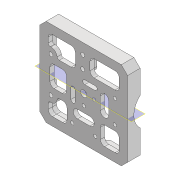
# Autodesk Inventor part: base_shell_2
Saved by Autodesk Inventor 2020 (Build 240168000, 168)
## iProperties
Created: 2022-01-22
Part Number: base_shell_2
Material: Generic
Document SubType Name: Modeling
Designer: Shuang Peng
Density: 1 g/cm^3
Appearance: Default
Author: Shuang Peng
Autodesk Inventor part; units mm, degrees
ref_plane "YZ Plane" through (0, 0, 0) normal (1, 0, 0) x (0, 1, 0)
ref_plane "XZ Plane" through (0, 0, 0) normal (0, 1, 0) x (-1, 0, 0)
ref_plane "XY Plane" through (0, 0, 0) normal (0, 0, 1) x (1, 0, 0)
sketch "Sketch1" plane through (0, 0, 0) normal (0, 0, 1) x (1, 0, 0)
  circle A0 centre (7.5, 4) radius 0.75 projected
  circle A1 centre (13, -5.9) radius 0.75 projected
  circle A2 centre (2, -5.9) radius 0.75 projected
  line L0 (15, -7) -> (15, 0) projected
  line L1 (11, 0) -> (15, 0) projected
  arc A3 (10, 1) -> (11, 0) centre (11, 1) ccw projected
  line L2 (10, 1) -> (10, 5) projected
  line L3 (6, 6) -> (9, 6) projected
  line L4 (5, 1) -> (5, 5) projected
  arc A4 (4, 0) -> (5, 1) centre (4, 1) ccw projected
  line L5 (0, 0) -> (4, 0) projected
  line L6 (0, -7) -> (0, 0) projected
  line L7 (1.5, -8.5) -> (5, -8.5) projected
  line L8 (13, -5.9) -> (2, -5.9)
  line L9 (7.5, -5.9) -> (7.5, -9.9)
  line L10 (7.5, -9.9) -> (-2.5, -9.9)
  line L11 (-23.5, -30.9) -> (-23.5, 11.1)
  line L12 (-23.5, 11.1) -> (18.5, 11.1)
  line L13 (18.5, 11.1) -> (18.5, -30.9)
  line L14 (18.5, -30.9) -> (-23.5, -30.9)
  line L15 (-23.5, -30.9) -> (18.5, 11.1) construction
  line L16 (-23.5, 11.1) -> (18.5, -30.9) construction
  circle A5 centre (-15.2, -15.4) radius 0.75 projected
  circle A6 centre (-15.2, -4.4) radius 0.75 projected
  circle A7 centre (-15.2, -15.4) radius 0.85
  circle A8 centre (-15.2, -4.4) radius 0.85
  circle A9 centre (-5.3, -9.9) radius 0.75 projected
  circle A10 centre (-5.3, -9.9) radius 0.85
  circle A11 centre (2, -5.9) radius 0.85
  circle A12 centre (13, -5.9) radius 0.85
  circle A13 centre (7.5, 4) radius 0.85
  line L17 (6, -7.5) -> (6, -4.5) projected
  arc A14 (9, -4.5) -> (6, -4.5) centre (7.5, -4.5) ccw projected
  line L18 (9, -4.5) -> (9, -7.5) projected
  line L19 (10, -8.5) -> (13.5, -8.5) projected
  arc A15 (6, 6) -> (5, 5) centre (6, 5) ccw projected
  line L20 (1.5, -8.5) -> (0, -7) projected
  arc A16 (5, -8.5) -> (6, -7.5) centre (5, -7.5) ccw projected
  arc A17 (9, -7.5) -> (10, -8.5) centre (10, -7.5) ccw projected
  line L21 (15, -7) -> (13.5, -8.5) projected
  arc A18 (10, 5) -> (9, 6) centre (9, 5) ccw projected
  dimension "d0" = 4
  dimension "d1" = 10
  dimension "d2" = 42
  dimension "d3" = 42
  dimension "d4" = 1.7
  dimension "d5" = 1.7
  dimension "d6" = 1.7
  dimension "d7" = 1.7
  dimension "d8" = 1.7
  dimension "d9" = 1.7
  constraints: 18 end point, 6 centre point, 6 coincident, 3 midpoint, 3 perpendicular, 2 parallel, 1 horizontal, 1 vertical
  measures "d0" distance of L9.start L9.end
  measures "d1" distance of L9.end L10.end
  measures "d2" distance of L11.start L11.end
  measures "d3" distance of L11.end L12.end
  measures "d4" diameter of A7
  measures "d5" diameter of A8
  measures "d6" diameter of A10
  measures "d7" diameter of A11
  measures "d8" diameter of A12
  measures "d9" diameter of A13
extrude "Extrusion1" add sketch "Sketch1" along normal blind 2 contours L21 L19 A17 L18 A14 L17 A16 L7 L20 L6 L5 A4 L4 A15 L3 A18 L2 A3 L1 L0 | L8 L17 A14 L18 | L11 L12 L13 L14
sketch "Sketch2" plane through (0, 0, 0) normal (0, 0, -1) x (-1, 0, 0)
  line L0 (23.5, -30.9) -> (-18.5, -30.9) projected
  line L1 (23.5, 11.1) -> (23.5, -30.9) projected
  line L2 (-18.5, 11.1) -> (23.5, 11.1) projected
  line L3 (-18.5, -30.9) -> (-18.5, 11.1) projected
  circle A0 centre (-2, -5.9) radius 0.85 projected
  circle A1 centre (15.2, -15.4) radius 0.85 projected
  circle A2 centre (15.2, -4.4) radius 0.85 projected
  circle A3 centre (5.3, -9.9) radius 0.85 projected
  circle A4 centre (-13, -5.9) radius 0.85 projected
  circle A5 centre (-7.5, 4) radius 0.85 projected
  line L4 (23.5, -30.9) -> (-18.5, -30.9) projected
  line L5 (-18.5, -30.9) -> (23.5, 11.1)
  line L6 (23.5, -30.9) -> (-18.5, 11.1)
  line L7 (-16.5, -28.9) -> (-16.5, 9.1)
  line L8 (-16.5, 9.1) -> (21.5, 9.1)
  line L9 (21.5, 9.1) -> (21.5, -28.9)
  line L10 (21.5, -28.9) -> (-16.5, -28.9)
  line L11 (-16.5, -28.9) -> (21.5, 9.1) construction
  line L12 (-16.5, 9.1) -> (21.5, -28.9) construction
  point P0 (0, 0)
  point P1 (2.5, -9.9)
  dimension "d12" = 38
  dimension "d13" = 38
  constraints: 16 end point, 3 midpoint, 2 parallel, 1 perpendicular, 1 vertical
  measures "d12" distance of L8.end L9.end
  measures "d13" distance of L7.end L8.end
extrude "Extrusion2" add sketch "Sketch2" along normal blind 4 contours L6 L9 L5 L1 | L0 L5 L10 L6 | L3 L6 L7 L5 | L5 L8 L6 L2
fillet "Fillet1" radius 2 1 edges at (16.5, -28.9, -2)
sketch "Sketch4" plane through (-23.5, -30.9, 2) normal (-1, 0, 0) x (0, 0, 1)
  circle A0 centre (-12, 21) radius 0.75 projected
  circle A1 centre (-12, 21) radius 9
  point P0 (-2, 30.9)
  dimension "d21" = 18
  constraints: 1 centre point, 1 coincident
  measures "d21" diameter of A1
extrude "Extrusion4" cut sketch "Sketch4" against normal blind 4
chamfer "Chamfer1" distance 3 angle 45 4 edges at (-23.5, -30.9, -1) (-23.5, 11.1, -1) (18.5, 11.1, -1) (18.5, -30.9, -1)
sketch "Sketch8" plane through (0, 0, 0) normal (0, 0, -1) x (-1, 0, 0)
  circle A0 centre (-2, -5.9) radius 0.85 projected
  circle A1 centre (15.2, -15.4) radius 0.85 projected
  circle A2 centre (15.2, -4.4) radius 0.85 projected
  circle A3 centre (5.3, -9.9) radius 0.85 projected
  circle A4 centre (-13, -5.9) radius 0.85 projected
  circle A5 centre (-7.5, 4) radius 0.85 projected
  line L0 (15.2, -4.4) -> (18.2, -4.4)
  line L1 (18.2, -4.4) -> (18.2, -1.4)
  line L2 (15.2, -15.4) -> (18.2, -15.4)
  line L3 (18.2, -15.4) -> (18.2, -18.4)
  circle A6 centre (18.2, -1.4) radius 0.95
  circle A7 centre (18.2, -18.4) radius 0.95
  line L4 (-14.5, -28.9) -> (21.5, -28.9) projected
  line L5 (21.5, -28.9) -> (21.5, 9.1) projected
  line L6 (21.5, 9.1) -> (-16.5, 9.1) projected
  line L7 (-16.5, 9.1) -> (-16.5, -26.9) projected
  arc A8 (-16.5, -26.9) -> (-14.5, -28.9) centre (-14.5, -26.9) ccw projected
  point P0 (0, 0)
  dimension "d53" = 3
  dimension "d54" = 3
  dimension "d55" = 3
  dimension "d56" = 3
  dimension "d57" = 1.9
  dimension "d58" = 1.9
  constraints: 8 end point, 2 centre point, 2 coincident, 2 horizontal, 2 perpendicular
  measures "d53" distance of L0.start L0.end
  measures "d54" distance of L0.end L1.end
  measures "d55" distance of L2.start L2.end
  measures "d56" distance of L2.end L3.end
  measures "d57" diameter of A6
  measures "d58" diameter of A7
extrude "Extrusion8" cut sketch "Sketch8" against normal blind 4 contours A6 | A7
sketch "Sketch9" plane through (0, 0, 0) normal (0, 0, -1) x (-1, 0, 0)
  circle A0 centre (18.2, -18.4) radius 0.95 projected
  circle A1 centre (18.2, -1.4) radius 0.95 projected
  circle A2 centre (-2, -5.9) radius 0.85 projected
  circle A3 centre (15.2, -15.4) radius 0.85 projected
  circle A4 centre (15.2, -4.4) radius 0.85 projected
  circle A5 centre (5.3, -9.9) radius 0.85 projected
  circle A6 centre (-13, -5.9) radius 0.85 projected
  circle A7 centre (-7.5, 4) radius 0.85 projected
  line L0 (0, 0) -> (3, 0)
  line L1 (3, 0) -> (3, 6)
  circle A8 centre (3, 6) radius 0.95
  circle A9 centre (3, 0) radius 0.95
  line L2 (-14.5, -28.9) -> (21.5, -28.9) projected
  line L3 (21.5, -28.9) -> (21.5, 9.1) projected
  line L4 (21.5, 9.1) -> (-16.5, 9.1) projected
  line L5 (-16.5, 9.1) -> (-16.5, -26.9) projected
  arc A10 (-16.5, -26.9) -> (-14.5, -28.9) centre (-14.5, -26.9) ccw projected
  dimension "d61" = 3
  dimension "d62" = 6
  dimension "d63" = 1.9
  dimension "d64" = 1.9
  constraints: 4 end point, 2 centre point, 2 coincident, 1 horizontal, 1 vertical
  measures "d61" distance of L0.start L0.end
  measures "d62" distance of L0.end L1.end
  measures "d63" diameter of A8
  measures "d64" diameter of A9
extrude "Extrusion9" cut sketch "Sketch9" against normal blind 4 contours A9 L1 L0 | L0 L1 A9 | A8
sketch "Sketch10" plane through (0, 0, 0) normal (0, 0, -1) x (-1, 0, 0)
  circle A0 centre (3, 0) radius 0.95 projected
  circle A1 centre (3, 6) radius 0.95 projected
  circle A2 centre (18.2, -18.4) radius 0.95 projected
  circle A3 centre (18.2, -1.4) radius 0.95 projected
  circle A4 centre (-2, -5.9) radius 0.85 projected
  circle A5 centre (15.2, -15.4) radius 0.85 projected
  circle A6 centre (15.2, -4.4) radius 0.85 projected
  circle A7 centre (5.3, -9.9) radius 0.85 projected
  circle A8 centre (-13, -5.9) radius 0.85 projected
  circle A9 centre (-7.5, 4) radius 0.85 projected
  line L0 (3, 0) -> (3, 6) construction
  line L1 (5.3, 0) -> (5.3, 6)
  line L2 (0.7, 6) -> (0.7, 0)
  arc A10 (0.7, 0) -> (5.3, 0) centre (3, 0) ccw
  arc A11 (5.3, 6) -> (0.7, 6) centre (3, 6) ccw
  line L3 (0.7, 6) -> (5.3, 6)
  line L4 (5.3, 6) -> (5.3, 10)
  line L5 (5.3, 10) -> (0.7, 10)
  line L6 (0.7, 10) -> (0.7, 6)
  line L7 (-14.5, -28.9) -> (21.5, -28.9) projected
  line L8 (21.5, -28.9) -> (21.5, 9.1) projected
  line L9 (21.5, 9.1) -> (-16.5, 9.1) projected
  line L10 (-16.5, 9.1) -> (-16.5, -26.9) projected
  arc A12 (-16.5, -26.9) -> (-14.5, -28.9) centre (-14.5, -26.9) ccw projected
  point P0 (0, 0)
  point P1 (3, 3)
  dimension "d67" = 4.6
  dimension "d68" = 4.6
  dimension "d69" = 4
  constraints: 16 end point, 4 point on circle, 4 tangent, 3 parallel, 2 centre point, 1 horizontal, 1 midpoint, 1 perpendicular, 1 vertical
  measures "d67" diameter of A11
  measures "d68" distance of L5.end L4.end
  measures "d69" distance of L4.end L3.end
extrude "Extrusion10" add sketch "Sketch10" along normal blind 2.5 contours L3 L1 A10 L2 A1 | A1 L3 A11 | A11 L6 L9 L4 | L9 L6 L5 L4
sketch "Sketch11" plane through (0, 0, 0) normal (0, 0, -1) x (-1, 0, 0)
  circle A0 centre (-7.5, 4) radius 0.85 projected
  circle A1 centre (-13, -5.9) radius 0.85 projected
  circle A2 centre (5.3, -9.9) radius 0.85 projected
  circle A3 centre (15.2, -4.4) radius 0.85 projected
  circle A4 centre (15.2, -15.4) radius 0.85 projected
  circle A5 centre (-2, -5.9) radius 0.85 projected
  line L0 (5.3, 9.1) -> (5.3, 0) projected
  arc A6 (0.7, 0) -> (5.3, 0) centre (3, 0) ccw projected
  line L1 (0.7, 0) -> (0.7, 9.1) projected
  line L2 (0.7, 9.1) -> (-16.5, 9.1) projected
  line L3 (-16.5, 9.1) -> (-16.5, -26.9) projected
  arc A7 (-16.5, -26.9) -> (-14.5, -28.9) centre (-14.5, -26.9) ccw projected
  line L4 (-14.5, -28.9) -> (21.5, -28.9) projected
  line L5 (21.5, -28.9) -> (21.5, 9.1) projected
  line L6 (21.5, 9.1) -> (5.3, 9.1) projected
  circle A8 centre (18.2, -1.4) radius 0.95 projected
  circle A9 centre (18.2, -18.4) radius 0.95 projected
  point P0 (0, 0)
extrude "Extrusion11" add sketch "Sketch11" against normal up to surface (2 mm away) contours A0 | A1 | A2 | A3 | A4 | A5
sketch "Sketch12" plane through (0, 0, 2) normal (0, 0, 1) x (1, 0, 0)
  arc A0 (0.5, -11.4) -> (1.5, -12.4) centre (1.5, -11.4) ccw projected
  line L0 (5, -12.4) -> (1.5, -12.4) projected
  arc A1 (6.5, -13.9) -> (5, -12.4) centre (5, -13.9) ccw projected
  line L1 (6.5, -17.4) -> (6.5, -13.9) projected
  line L2 (13.5, -17.4) -> (6.5, -17.4) projected
  line L3 (15, -15.9) -> (13.5, -17.4) projected
  line L4 (15, -15.9) -> (15, -12.4) projected
  arc A2 (15, -12.4) -> (14, -11.4) centre (14, -12.4) ccw projected
  line L5 (14, -11.4) -> (11, -11.4) projected
  arc A3 (11, -8.4) -> (11, -11.4) centre (11, -9.9) ccw projected
  line L6 (11, -8.4) -> (14, -8.4) projected
  arc A4 (14, -8.4) -> (15, -7.4) centre (14, -7.4) ccw projected
  line L7 (15, -7.4) -> (15, -3.9) projected
  line L8 (13.5, -2.4) -> (15, -3.9) projected
  line L9 (13.5, -2.4) -> (6.5, -2.4) projected
  line L10 (6.5, -5.9) -> (6.5, -2.4) projected
  arc A5 (5, -7.4) -> (6.5, -5.9) centre (5, -5.9) ccw projected
  line L11 (5, -7.4) -> (1.5, -7.4) projected
  arc A6 (1.5, -7.4) -> (0.5, -8.4) centre (1.5, -8.4) ccw projected
  line L12 (0.5, -11.4) -> (0.5, -8.4) projected
  circle A7 centre (12.4, -15.4) radius 0.725 projected
  circle A8 centre (12.4, -4.4) radius 0.725 projected
  circle A9 centre (2.5, -9.9) radius 0.725 projected
  arc A10 (-4, -12.9) -> (-5, -13.9) centre (-4, -13.9) ccw projected
  line L13 (-5, -17.4) -> (-5, -13.9) projected
  arc A11 (-6.5, -18.9) -> (-5, -17.4) centre (-6.5, -17.4) ccw projected
  line L14 (-10, -18.9) -> (-6.5, -18.9) projected
  line L15 (-10, -25.9) -> (-10, -18.9) projected
  line L16 (-8.5, -27.4) -> (-10, -25.9) projected
  line L17 (-8.5, -27.4) -> (-5, -27.4) projected
  arc A12 (-5, -27.4) -> (-4, -26.4) centre (-5, -26.4) ccw projected
  line L18 (-4, -26.4) -> (-4, -23.4) projected
  arc A13 (-1, -23.4) -> (-4, -23.4) centre (-2.5, -23.4) ccw projected
  line L19 (-1, -23.4) -> (-1, -26.4) projected
  arc A14 (-1, -26.4) -> (0, -27.4) centre (0, -26.4) ccw projected
  line L20 (0, -27.4) -> (3.5, -27.4) projected
  line L21 (5, -25.9) -> (3.5, -27.4) projected
  line L22 (5, -25.9) -> (5, -18.9) projected
  line L23 (1.5, -18.9) -> (5, -18.9) projected
  arc A15 (0, -17.4) -> (1.5, -18.9) centre (1.5, -17.4) ccw projected
  line L24 (0, -17.4) -> (0, -13.9) projected
  arc A16 (0, -13.9) -> (-1, -12.9) centre (-1, -13.9) ccw projected
  line L25 (-4, -12.9) -> (-1, -12.9) projected
  circle A17 centre (-8, -24.8) radius 0.725 projected
  circle A18 centre (3, -24.8) radius 0.725 projected
  circle A19 centre (-2.5, -14.9) radius 0.725 projected
  point P0 (0, 0)
hole "Hole1" at (12.4, -4.4, 2) at (12.4, -15.4, 2) at (2.5, -9.9, 2) at (-2.5, -14.9, 2) at (-8, -24.8, 2) at (3, -24.8, 2) direction (0, 0, -1) diameter 1.6 depth 10
sketch "Sketch13" plane through (0, 0, 2) normal (0, 0, 1) x (1, 0, 0)
  circle A0 centre (-8, -24.8) radius 0.8 projected
  circle A1 centre (2.5, -9.9) radius 0.8 projected
  circle A2 centre (12.4, -4.4) radius 0.8 projected
  circle A3 centre (12.4, -15.4) radius 0.8 projected
  circle A4 centre (-2.5, -14.9) radius 0.8 projected
  circle A5 centre (3, -24.8) radius 0.8 projected
  circle A6 centre (-3, 0) radius 0.95 projected
  circle A7 centre (-3, 6) radius 0.95 projected
  circle A8 centre (-18.2, -18.4) radius 0.95 projected
  circle A9 centre (-18.2, -1.4) radius 0.95 projected
  line L0 (18.5, -27.9) -> (15.5, -30.9) projected
  line L1 (18.5, -27.9) -> (18.5, 8.1) projected
  line L2 (15.5, 11.1) -> (18.5, 8.1) projected
  line L3 (15.5, 11.1) -> (-20.5, 11.1) projected
  line L4 (-23.5, 8.1) -> (-20.5, 11.1) projected
  line L5 (-23.5, 8.1) -> (-23.5, -27.9) projected
  line L6 (-20.5, -30.9) -> (-23.5, -27.9) projected
  line L7 (-20.5, -30.9) -> (15.5, -30.9) projected
  circle A10 centre (12.4, -4.4) radius 0.8 projected
  line L8 (12.4, -4.4) -> (12.4, -15.4)
  circle A11 centre (2.5, -9.9) radius 0.8 projected
  line L9 (2.5, -9.9) -> (12.4, -9.9)
  line L10 (7.45, -6.9) -> (7.45, -12.9) construction
  line L11 (5.45, -6.9) -> (5.45, -12.9)
  line L12 (9.45, -12.9) -> (9.45, -6.9)
  arc A12 (9.45, -6.9) -> (5.45, -6.9) centre (7.45, -6.9) ccw
  arc A13 (5.45, -12.9) -> (9.45, -12.9) centre (7.45, -12.9) ccw
  circle A14 centre (3, -24.8) radius 0.8 projected
  circle A15 centre (-8, -24.8) radius 0.8 projected
  line L13 (3, -24.8) -> (-8, -24.8)
  circle A16 centre (-2.5, -14.9) radius 0.8 projected
  line L14 (-2.5, -14.9) -> (-2.5, -24.8)
  line L15 (0.5, -19.85) -> (-5.5, -19.85) construction
  line L16 (0.5, -17.85) -> (-5.5, -17.85)
  line L17 (-5.5, -21.85) -> (0.5, -21.85)
  arc A17 (0.5, -21.85) -> (0.5, -17.85) centre (0.5, -19.85) ccw
  arc A18 (-5.5, -17.85) -> (-5.5, -21.85) centre (-5.5, -19.85) ccw
  point P0 (0, 0)
  point P1 (7.45, -9.9)
  point P2 (-2.5, -19.85)
  dimension "d82" = 3
  dimension "d83" = 4
  dimension "d84" = 3
  dimension "d85" = 4
  constraints: 24 end point, 8 point on circle, 8 tangent, 6 midpoint, 4 centre point, 2 parallel, 2 perpendicular, 1 horizontal, 1 vertical
  measures "d82" distance of point (7.45, -9.9) L10.end
  measures "d83" diameter of A13
  measures "d84" distance of point (-2.5, -19.85) L15.end
  measures "d85" diameter of A18
extrude "Extrusion12" cut sketch "Sketch13" against normal blind 10 contours L11 A12 L12 L9 | L9 L12 A13 L11 | L16 A17 L17 L14 | L14 L17 A18 L16
sketch "Sketch14" plane through (18.5, -27.9, -4) normal (1, 0, 0) x (0, 0, -1)
  circle A0 centre (6, 18) radius 1 projected
  circle A1 centre (6, 18) radius 9
  line L0 (0, 0) -> (-6, 0) projected
  line L1 (0, 36) -> (0, 0) projected
  line L2 (-6, 36) -> (0, 36) projected
  line L3 (-6, 0) -> (-6, 36) projected
  point P0 (-4, 27.9)
  point P1 (0, 11.2918)
  point P2 (0, 24.7082)
  dimension "d88" = 18
  constraints: 1 centre point, 1 coincident
  measures "d88" diameter of A1
extrude "Extrusion13" cut sketch "Sketch14" against normal blind 10 contours L1 A1 picked at (-0.4747, 16.3042)
sketch "Sketch15" plane through (-20.5, -30.9, 2) normal (0, -1, 0) x (1, 0, 0)
  line L0 (36, 0) -> (36, -6) projected
  line L1 (0, 0) -> (36, 0) projected
  line L2 (0, -6) -> (0, 0) projected
  line L3 (36, -6) -> (0, -6) projected
  circle A0 centre (18, -12) radius 1 projected
  circle A1 centre (18, -12) radius 9
  point P0 (20.5, -2)
  point P1 (11.2918, -6)
  point P2 (24.7082, -6)
  dimension "d91" = 18
  constraints: 1 centre point, 1 coincident
  measures "d91" diameter of A1
extrude "Extrusion14" cut sketch "Sketch15" against normal blind 10 contours L3 A1 picked at (17.6404, -5.0216)
fillet "Fillet5" radius 2 3 edges at (-21.5, 9.1, -2) (-21.5, -28.9, -2) (16.5, 9.1, -2)
sketch "Sketch16" plane through (0, 0, 0) normal (0, 0, -1) x (-1, 0, 0)
  arc A0 (-14.5, 9.1) -> (-16.5, 7.1) centre (-14.5, 7.1) ccw projected
  line L0 (-16.5, 7.1) -> (-16.5, -26.9) projected
  arc A1 (-16.5, -26.9) -> (-14.5, -28.9) centre (-14.5, -26.9) ccw projected
  line L1 (-14.5, -28.9) -> (19.5, -28.9) projected
  arc A2 (19.5, -28.9) -> (21.5, -26.9) centre (19.5, -26.9) ccw projected
  line L2 (21.5, -26.9) -> (21.5, 7.1) projected
  arc A3 (21.5, 7.1) -> (19.5, 9.1) centre (19.5, 7.1) ccw projected
  line L3 (19.5, 9.1) -> (5.3, 9.1) projected
  line L4 (5.3, 9.1) -> (5.3, 0) projected
  arc A4 (0.7, 0) -> (5.3, 0) centre (3, 0) ccw projected
  line L5 (0.7, 0) -> (0.7, 9.1) projected
  line L6 (0.7, 9.1) -> (-14.5, 9.1) projected
  circle A5 centre (18.2, -1.4) radius 0.95 projected
  circle A6 centre (18.2, -18.4) radius 0.95 projected
  circle A7 centre (-3, -24.8) radius 0.8 projected
  circle A8 centre (2.5, -14.9) radius 0.8 projected
  circle A9 centre (-12.4, -15.4) radius 0.8 projected
  circle A10 centre (-12.4, -4.4) radius 0.8 projected
  circle A11 centre (-2.5, -9.9) radius 0.8 projected
  circle A12 centre (8, -24.8) radius 0.8 projected
  line L7 (-5.45, -6.9) -> (-5.45, -12.9) projected
  arc A13 (-9.45, -12.9) -> (-5.45, -12.9) centre (-7.45, -12.9) ccw projected
  line L8 (-9.45, -12.9) -> (-9.45, -6.9) projected
  arc A14 (-5.45, -6.9) -> (-9.45, -6.9) centre (-7.45, -6.9) ccw projected
  line L9 (-0.5, -17.85) -> (5.5, -17.85) projected
  arc A15 (5.5, -21.85) -> (5.5, -17.85) centre (5.5, -19.85) ccw projected
  line L10 (5.5, -21.85) -> (-0.5, -21.85) projected
  arc A16 (-0.5, -17.85) -> (-0.5, -21.85) centre (-0.5, -19.85) ccw projected
  line L11 (-12.5, -26.9) -> (-7.5, -26.9)
  line L12 (-5.5, -24.9) -> (-5.5, -19.9)
  line L13 (-7.5, -17.9) -> (-12.5, -17.9)
  line L14 (-14.5, -19.9) -> (-14.5, -24.9)
  arc A17 (-5.5, -19.9) -> (-7.5, -17.9) centre (-7.5, -19.9) ccw
  arc A18 (-7.5, -26.9) -> (-5.5, -24.9) centre (-7.5, -24.9) ccw
  arc A19 (-14.5, -24.9) -> (-12.5, -26.9) centre (-12.5, -24.9) ccw
  arc A20 (-12.5, -17.9) -> (-14.5, -19.9) centre (-12.5, -19.9) ccw
  point P0 (0, 0)
  point P1 (-5.5, -17.9)
  point P2 (-5.5, -26.9)
  point P3 (-14.5, -17.9)
  dimension "d95" = 9
  dimension "d96" = 9
  dimension "d97" = 2
  constraints: 8 end point, 8 point on circle, 8 point on line, 8 tangent, 4 centre point, 3 equal radius, 2 parallel, 1 horizontal, 1 perpendicular
  measures "d95" distance of point (-14.5, -17.9) point (-5.5, -17.9)
  measures "d96" distance of point (-5.5, -17.9) point (-5.5, -26.9)
  measures "d97" radius of A17
extrude "Extrusion15" cut sketch "Sketch16" against normal blind 10 contours A19 L14 A20 L13 A17 L12 A18 L11
sketch "Sketch17" plane through (0, 0, 0) normal (0, 0, -1) x (-1, 0, 0)
  line L0 (-12.5, -17.9) -> (-7.5, -17.9) projected
  arc A0 (-5.5, -19.9) -> (-7.5, -17.9) centre (-7.5, -19.9) ccw projected
  line L1 (-5.5, -19.9) -> (-5.5, -24.9) projected
  arc A1 (-7.5, -26.9) -> (-5.5, -24.9) centre (-7.5, -24.9) ccw projected
  line L2 (-7.5, -26.9) -> (-12.5, -26.9) projected
  arc A2 (-14.5, -24.9) -> (-12.5, -26.9) centre (-12.5, -24.9) ccw projected
  line L3 (-14.5, -24.9) -> (-14.5, -19.9) projected
  arc A3 (-12.5, -17.9) -> (-14.5, -19.9) centre (-12.5, -19.9) ccw projected
  arc A4 (-14.5, 9.1) -> (-16.5, 7.1) centre (-14.5, 7.1) ccw projected
  line L4 (-16.5, 7.1) -> (-16.5, -26.9) projected
  arc A5 (-16.5, -26.9) -> (-14.5, -28.9) centre (-14.5, -26.9) ccw projected
  line L5 (-14.5, -28.9) -> (19.5, -28.9) projected
  arc A6 (19.5, -28.9) -> (21.5, -26.9) centre (19.5, -26.9) ccw projected
  line L6 (21.5, -26.9) -> (21.5, 7.1) projected
  arc A7 (21.5, 7.1) -> (19.5, 9.1) centre (19.5, 7.1) ccw projected
  line L7 (19.5, 9.1) -> (5.3, 9.1) projected
  line L8 (5.3, 9.1) -> (5.3, 0) projected
  arc A8 (0.7, 0) -> (5.3, 0) centre (3, 0) ccw projected
  line L9 (0.7, 0) -> (0.7, 9.1) projected
  line L10 (0.7, 9.1) -> (-14.5, 9.1) projected
  circle A9 centre (18.2, -1.4) radius 0.95 projected
  circle A10 centre (18.2, -18.4) radius 0.95 projected
  circle A11 centre (-3, -24.8) radius 0.8 projected
  circle A12 centre (2.5, -14.9) radius 0.8 projected
  circle A13 centre (-12.4, -15.4) radius 0.8 projected
  circle A14 centre (-12.4, -4.4) radius 0.8 projected
  circle A15 centre (-2.5, -9.9) radius 0.8 projected
  circle A16 centre (8, -24.8) radius 0.8 projected
  line L11 (-5.45, -6.9) -> (-5.45, -12.9) projected
  arc A17 (-9.45, -12.9) -> (-5.45, -12.9) centre (-7.45, -12.9) ccw projected
  line L12 (-9.45, -12.9) -> (-9.45, -6.9) projected
  arc A18 (-5.45, -6.9) -> (-9.45, -6.9) centre (-7.45, -6.9) ccw projected
  line L13 (-0.5, -17.85) -> (5.5, -17.85) projected
  arc A19 (5.5, -21.85) -> (5.5, -17.85) centre (5.5, -19.85) ccw projected
  line L14 (5.5, -21.85) -> (-0.5, -21.85) projected
  arc A20 (-0.5, -17.85) -> (-0.5, -21.85) centre (-0.5, -19.85) ccw projected
  line L15 (21.5, -16.6082) -> (21.5, -3.1918) projected
  line L16 (21.5, -9.9) -> (-16.5, -9.9)
  line L17 (-16.5, -3.1918) -> (-16.5, -16.6082) projected
  circle A21 centre (2.5, -9.9) radius 1.5
  point P0 (0, 0)
  dimension "d100" = 3
  constraints: 3 midpoint, 2 end point, 1 centre point
  measures "d100" diameter of A21
extrude "Extrusion16" cut sketch "Sketch17" against normal blind 10 contours A21 L16 | L16 A21
sketch "Sketch18" plane through (0, 0, 0) normal (0, 0, -1) x (-1, 0, 0)
  circle A0 centre (2.5, -9.9) radius 1.5 projected
  line L0 (-12.5, -17.9) -> (-7.5, -17.9) projected
  arc A1 (-5.5, -19.9) -> (-7.5, -17.9) centre (-7.5, -19.9) ccw projected
  line L1 (-5.5, -19.9) -> (-5.5, -24.9) projected
  arc A2 (-7.5, -26.9) -> (-5.5, -24.9) centre (-7.5, -24.9) ccw projected
  line L2 (-7.5, -26.9) -> (-12.5, -26.9) projected
  arc A3 (-14.5, -24.9) -> (-12.5, -26.9) centre (-12.5, -24.9) ccw projected
  line L3 (-14.5, -24.9) -> (-14.5, -19.9) projected
  arc A4 (-12.5, -17.9) -> (-14.5, -19.9) centre (-12.5, -19.9) ccw projected
  arc A5 (-14.5, 9.1) -> (-16.5, 7.1) centre (-14.5, 7.1) ccw projected
  line L4 (-16.5, 7.1) -> (-16.5, -26.9) projected
  arc A6 (-16.5, -26.9) -> (-14.5, -28.9) centre (-14.5, -26.9) ccw projected
  line L5 (-14.5, -28.9) -> (19.5, -28.9) projected
  arc A7 (19.5, -28.9) -> (21.5, -26.9) centre (19.5, -26.9) ccw projected
  line L6 (21.5, -26.9) -> (21.5, 7.1) projected
  arc A8 (21.5, 7.1) -> (19.5, 9.1) centre (19.5, 7.1) ccw projected
  line L7 (19.5, 9.1) -> (5.3, 9.1) projected
  line L8 (5.3, 9.1) -> (5.3, 0) projected
  arc A9 (0.7, 0) -> (5.3, 0) centre (3, 0) ccw projected
  line L9 (0.7, 0) -> (0.7, 9.1) projected
  line L10 (0.7, 9.1) -> (-14.5, 9.1) projected
  circle A10 centre (18.2, -1.4) radius 0.95 projected
  circle A11 centre (18.2, -18.4) radius 0.95 projected
  circle A12 centre (-3, -24.8) radius 0.8 projected
  circle A13 centre (2.5, -14.9) radius 0.8 projected
  circle A14 centre (-12.4, -15.4) radius 0.8 projected
  circle A15 centre (-12.4, -4.4) radius 0.8 projected
  circle A16 centre (-2.5, -9.9) radius 0.8 projected
  circle A17 centre (8, -24.8) radius 0.8 projected
  line L11 (-5.45, -6.9) -> (-5.45, -12.9) projected
  arc A18 (-9.45, -12.9) -> (-5.45, -12.9) centre (-7.45, -12.9) ccw projected
  line L12 (-9.45, -12.9) -> (-9.45, -6.9) projected
  arc A19 (-5.45, -6.9) -> (-9.45, -6.9) centre (-7.45, -6.9) ccw projected
  line L13 (-0.5, -17.85) -> (5.5, -17.85) projected
  arc A20 (5.5, -21.85) -> (5.5, -17.85) centre (5.5, -19.85) ccw projected
  line L14 (5.5, -21.85) -> (-0.5, -21.85) projected
  arc A21 (-0.5, -17.85) -> (-0.5, -21.85) centre (-0.5, -19.85) ccw projected
  line L15 (-2.5, -9.9) -> (-0.5, -9.9)
  line L16 (-0.5, -9.9) -> (-0.5, -4.9)
  line L17 (2, -4.9) -> (-3, -4.9) construction
  line L18 (2, -3.9) -> (-3, -3.9)
  line L19 (-3, -5.9) -> (2, -5.9)
  arc A22 (2, -5.9) -> (2, -3.9) centre (2, -4.9) ccw
  arc A23 (-3, -3.9) -> (-3, -5.9) centre (-3, -4.9) ccw
  circle A24 centre (2.5, -14.9) radius 0.8 projected
  line L20 (2.5, -14.9) -> (2.5, -12.9)
  line L21 (2.5, -12.9) -> (7.5, -12.9)
  line L22 (7.6461, -10.4) -> (7.6461, -15.4) construction
  line L23 (6.6461, -10.4) -> (6.6461, -15.4)
  line L24 (8.6461, -15.4) -> (8.6461, -10.4)
  arc A25 (8.6461, -10.4) -> (6.6461, -10.4) centre (7.6461, -10.4) ccw
  arc A26 (6.6461, -15.4) -> (8.6461, -15.4) centre (7.6461, -15.4) ccw
  point P0 (0, 0)
  point P1 (7.6461, -12.9)
  dimension "d103" = 2
  dimension "d104" = 5
  dimension "d105" = 2.5
  dimension "d106" = 2
  dimension "d107" = 2
  dimension "d108" = 5
  dimension "d109" = 2.5
  dimension "d110" = 2
  constraints: 24 end point, 8 point on circle, 8 tangent, 4 centre point, 2 horizontal, 2 midpoint, 2 parallel, 2 perpendicular, 2 vertical
  measures "d103" distance of L15.start L15.end
  measures "d104" distance of L15.end L16.end
  measures "d105" distance of L16.end L17.end
  measures "d106" diameter of A23
  measures "d107" distance of L20.start L20.end
  measures "d108" distance of L20.end L21.end
  measures "d109" distance of point (7.646, -12.9) L22.end
  measures "d110" diameter of A26
extrude "Extrusion17" cut sketch "Sketch18" against normal blind 10 contours A22 L19 A23 L18 | A25 L24 A26 L23
ref_plane "Work Plane1" through (-20.5, -9.9, 2) normal (0, -1, 0) x (1, 0, 0)
mirror "Mirror1" about plane through (-20.5, -9.9, 2) normal (0, -1, 0) of "Extrusion15"
thicken "Thicken1" operation add thickness 5 both sides no extend neighbours yes toward (-1, 0, 0) faces at (5.5, 3.4333, 0.6667)
thicken "Thicken2" operation add thickness 1 both sides no extend neighbours yes toward (0, 1, 0) faces at (9.1667, -1.9, 1.3333)
sketch "Sketch19" plane through (0, 0, 0) normal (0, 0, -1) x (-1, 0, 0)
  line L0 (-16.5, 7.1) -> (-16.5, -26.9) projected
  arc A0 (-16.5, -26.9) -> (-14.5, -28.9) centre (-14.5, -26.9) ccw projected
  line L1 (-14.5, -28.9) -> (19.5, -28.9) projected
  arc A1 (19.5, -28.9) -> (21.5, -26.9) centre (19.5, -26.9) ccw projected
  line L2 (21.5, -26.9) -> (21.5, 7.1) projected
  arc A2 (21.5, 7.1) -> (19.5, 9.1) centre (19.5, 7.1) ccw projected
  line L3 (19.5, 9.1) -> (5.3, 9.1) projected
  line L4 (5.3, 9.1) -> (5.3, 0) projected
  arc A3 (0.7, 0) -> (5.3, 0) centre (3, 0) ccw projected
  line L5 (0.7, 0) -> (0.7, 9.1) projected
  line L6 (0.7, 9.1) -> (-14.5, 9.1) projected
  arc A4 (-14.5, 9.1) -> (-16.5, 7.1) centre (-14.5, 7.1) ccw projected
  line L7 (-3, -3.9) -> (2, -3.9) projected
  arc A5 (2, -5.9) -> (2, -3.9) centre (2, -4.9) ccw projected
  line L8 (2, -5.9) -> (-3, -5.9) projected
  arc A6 (-3, -3.9) -> (-3, -5.9) centre (-3, -4.9) ccw projected
  line L9 (-14.5, 1.1) -> (-14.5, 5.1) projected
  arc A7 (-12.5, 7.1) -> (-14.5, 5.1) centre (-12.5, 5.1) ccw projected
  line L10 (-12.5, 7.1) -> (-2.5, 7.1) projected
  arc A8 (-0.5, 5.1) -> (-2.5, 7.1) centre (-2.5, 5.1) ccw projected
  line L11 (-0.5, 5.1) -> (-0.5, 1.1) projected
  arc A9 (-2.5, -0.9) -> (-0.5, 1.1) centre (-2.5, 1.1) ccw projected
  line L12 (-2.5, -0.9) -> (-12.5, -0.9) projected
  arc A10 (-14.5, 1.1) -> (-12.5, -0.9) centre (-12.5, 1.1) ccw projected
  line L13 (8.6461, -10.4) -> (8.6461, -15.4) projected
  arc A11 (6.6461, -15.4) -> (8.6461, -15.4) centre (7.6461, -15.4) ccw projected
  line L14 (6.6461, -15.4) -> (6.6461, -10.4) projected
  arc A12 (8.6461, -10.4) -> (6.6461, -10.4) centre (7.6461, -10.4) ccw projected
  circle A13 centre (2.5, -9.9) radius 1.5 projected
  line L15 (-12.5, -17.9) -> (-7.5, -17.9) projected
  arc A14 (-5.5, -19.9) -> (-7.5, -17.9) centre (-7.5, -19.9) ccw projected
  line L16 (-5.5, -19.9) -> (-5.5, -24.9) projected
  arc A15 (-7.5, -26.9) -> (-5.5, -24.9) centre (-7.5, -24.9) ccw projected
  line L17 (-7.5, -26.9) -> (-12.5, -26.9) projected
  arc A16 (-14.5, -24.9) -> (-12.5, -26.9) centre (-12.5, -24.9) ccw projected
  line L18 (-14.5, -24.9) -> (-14.5, -19.9) projected
  arc A17 (-12.5, -17.9) -> (-14.5, -19.9) centre (-12.5, -19.9) ccw projected
  circle A18 centre (18.2, -1.4) radius 0.95 projected
  circle A19 centre (18.2, -18.4) radius 0.95 projected
  circle A20 centre (-3, -24.8) radius 0.8 projected
  circle A21 centre (2.5, -14.9) radius 0.8 projected
  circle A22 centre (-12.4, -15.4) radius 0.8 projected
  circle A23 centre (-12.4, -4.4) radius 0.8 projected
  circle A24 centre (-2.5, -9.9) radius 0.8 projected
  circle A25 centre (8, -24.8) radius 0.8 projected
  line L19 (-5.45, -6.9) -> (-5.45, -12.9) projected
  arc A26 (-9.45, -12.9) -> (-5.45, -12.9) centre (-7.45, -12.9) ccw projected
  line L20 (-9.45, -12.9) -> (-9.45, -6.9) projected
  arc A27 (-5.45, -6.9) -> (-9.45, -6.9) centre (-7.45, -6.9) ccw projected
  line L21 (-0.5, -17.85) -> (5.5, -17.85) projected
  arc A28 (5.5, -21.85) -> (5.5, -17.85) centre (5.5, -19.85) ccw projected
  line L22 (5.5, -21.85) -> (-0.5, -21.85) projected
  arc A29 (-0.5, -17.85) -> (-0.5, -21.85) centre (-0.5, -19.85) ccw projected
  line L23 (17.5, -26.9) -> (12.5, -26.9)
  line L24 (10.5, -24.9) -> (10.5, -19.9)
  line L25 (12.5, -17.9) -> (19.5, -17.9)
  line L26 (19.5, -17.9) -> (19.5, -24.9)
  line L27 (18.2, -18.4) -> (22.2, -18.4) construction
  line L28 (18.2, -21.4) -> (22.2, -21.4)
  line L29 (22.2, -15.4) -> (18.2, -15.4)
  arc A30 (18.2, -15.4) -> (18.2, -21.4) centre (18.2, -18.4) ccw
  arc A31 (22.2, -21.4) -> (22.2, -15.4) centre (22.2, -18.4) ccw
  line L30 (15.2, -18.4) -> (15.2, -17.9)
  arc A32 (12.5, -17.9) -> (10.5, -19.9) centre (12.5, -19.9) ccw
  arc A33 (10.5, -24.9) -> (12.5, -26.9) centre (12.5, -24.9) ccw
  arc A34 (17.5, -26.9) -> (19.5, -24.9) centre (17.5, -24.9) ccw
  point P0 (0, 0)
  point P1 (10.5, -17.9)
  point P2 (10.5, -26.9)
  point P3 (20.2, -18.4)
  point P4 (19.5, -21.4)
  dimension "d117" = 9
  dimension "d118" = 9
  dimension "d119" = 4
  dimension "d120" = 6
  dimension "d121" = 2
  constraints: 18 end point, 11 point on circle, 11 tangent, 7 point on line, 5 centre point, 3 parallel, 2 equal radius, 2 horizontal, 2 perpendicular, 1 midpoint
  measures "d117" distance of point (10.5, -17.9) L25.end
  measures "d118" distance of point (10.5, -26.9) point (10.5, -17.9)
  measures "d119" distance of L27.start L27.end
  measures "d120" diameter of A31
  measures "d121" radius of A32
extrude "Extrusion18" cut sketch "Sketch19" against normal blind 10 contours L26 A34 L23 A33 L24 A32 L25 L30 A30 L28
fillet "Fillet6" radius 1 2 edges at (-19.5, -21.4, 1) (-15.2, -17.9, 1)
sketch "Sketch20" plane through (0, 0, 0) normal (0, 0, -1) x (-1, 0, 0)
  arc A0 (15.2235, -18.775) -> (14.2314, -17.9) centre (14.2314, -18.9) ccw projected
  arc A1 (15.2235, -18.775) -> (18.2, -21.4) centre (18.2, -18.4) ccw projected
  line L0 (18.2, -21.4) -> (18.5, -21.4) projected
  arc A2 (19.5, -22.4) -> (18.5, -21.4) centre (18.5, -22.4) ccw projected
  line L1 (19.5, -22.4) -> (19.5, -24.9) projected
  arc A3 (17.5, -26.9) -> (19.5, -24.9) centre (17.5, -24.9) ccw projected
  line L2 (17.5, -26.9) -> (12.5, -26.9) projected
  arc A4 (10.5, -24.9) -> (12.5, -26.9) centre (12.5, -24.9) ccw projected
  line L3 (10.5, -24.9) -> (10.5, -19.9) projected
  arc A5 (12.5, -17.9) -> (10.5, -19.9) centre (12.5, -19.9) ccw projected
  line L4 (12.5, -17.9) -> (14.2314, -17.9) projected
  line L5 (-16.5, 7.1) -> (-16.5, -26.9) projected
  arc A6 (-16.5, -26.9) -> (-14.5, -28.9) centre (-14.5, -26.9) ccw projected
  line L6 (-14.5, -28.9) -> (19.5, -28.9) projected
  arc A7 (19.5, -28.9) -> (21.5, -26.9) centre (19.5, -26.9) ccw projected
  line L7 (21.5, -26.9) -> (21.5, 7.1) projected
  arc A8 (21.5, 7.1) -> (19.5, 9.1) centre (19.5, 7.1) ccw projected
  line L8 (19.5, 9.1) -> (5.3, 9.1) projected
  line L9 (5.3, 9.1) -> (5.3, 0) projected
  arc A9 (0.7, 0) -> (5.3, 0) centre (3, 0) ccw projected
  line L10 (0.7, 0) -> (0.7, 9.1) projected
  line L11 (0.7, 9.1) -> (-14.5, 9.1) projected
  arc A10 (-14.5, 9.1) -> (-16.5, 7.1) centre (-14.5, 7.1) ccw projected
  line L12 (-3, -3.9) -> (2, -3.9) projected
  arc A11 (2, -5.9) -> (2, -3.9) centre (2, -4.9) ccw projected
  line L13 (2, -5.9) -> (-3, -5.9) projected
  arc A12 (-3, -3.9) -> (-3, -5.9) centre (-3, -4.9) ccw projected
  line L14 (-14.5, 1.1) -> (-14.5, 5.1) projected
  arc A13 (-12.5, 7.1) -> (-14.5, 5.1) centre (-12.5, 5.1) ccw projected
  line L15 (-12.5, 7.1) -> (-2.5, 7.1) projected
  arc A14 (-0.5, 5.1) -> (-2.5, 7.1) centre (-2.5, 5.1) ccw projected
  line L16 (-0.5, 5.1) -> (-0.5, 1.1) projected
  arc A15 (-2.5, -0.9) -> (-0.5, 1.1) centre (-2.5, 1.1) ccw projected
  line L17 (-2.5, -0.9) -> (-12.5, -0.9) projected
  arc A16 (-14.5, 1.1) -> (-12.5, -0.9) centre (-12.5, 1.1) ccw projected
  line L18 (8.6461, -10.4) -> (8.6461, -15.4) projected
  arc A17 (6.6461, -15.4) -> (8.6461, -15.4) centre (7.6461, -15.4) ccw projected
  line L19 (6.6461, -15.4) -> (6.6461, -10.4) projected
  arc A18 (8.6461, -10.4) -> (6.6461, -10.4) centre (7.6461, -10.4) ccw projected
  circle A19 centre (2.5, -9.9) radius 1.5 projected
  line L20 (-12.5, -17.9) -> (-7.5, -17.9) projected
  arc A20 (-5.5, -19.9) -> (-7.5, -17.9) centre (-7.5, -19.9) ccw projected
  line L21 (-5.5, -19.9) -> (-5.5, -24.9) projected
  arc A21 (-7.5, -26.9) -> (-5.5, -24.9) centre (-7.5, -24.9) ccw projected
  line L22 (-7.5, -26.9) -> (-12.5, -26.9) projected
  arc A22 (-14.5, -24.9) -> (-12.5, -26.9) centre (-12.5, -24.9) ccw projected
  line L23 (-14.5, -24.9) -> (-14.5, -19.9) projected
  arc A23 (-12.5, -17.9) -> (-14.5, -19.9) centre (-12.5, -19.9) ccw projected
  circle A24 centre (18.2, -1.4) radius 0.95 projected
  circle A25 centre (18.2, -18.4) radius 0.95 projected
  circle A26 centre (-3, -24.8) radius 0.8 projected
  circle A27 centre (2.5, -14.9) radius 0.8 projected
  circle A28 centre (-12.4, -15.4) radius 0.8 projected
  circle A29 centre (-12.4, -4.4) radius 0.8 projected
  circle A30 centre (-2.5, -9.9) radius 0.8 projected
  circle A31 centre (8, -24.8) radius 0.8 projected
  line L24 (-5.45, -6.9) -> (-5.45, -12.9) projected
  arc A32 (-9.45, -12.9) -> (-5.45, -12.9) centre (-7.45, -12.9) ccw projected
  line L25 (-9.45, -12.9) -> (-9.45, -6.9) projected
  arc A33 (-5.45, -6.9) -> (-9.45, -6.9) centre (-7.45, -6.9) ccw projected
  line L26 (-0.5, -17.85) -> (5.5, -17.85) projected
  arc A34 (5.5, -21.85) -> (5.5, -17.85) centre (5.5, -19.85) ccw projected
  line L27 (5.5, -21.85) -> (-0.5, -21.85) projected
  arc A35 (-0.5, -17.85) -> (-0.5, -21.85) centre (-0.5, -19.85) ccw projected
  line L28 (17.5, 7.1) -> (8.5, 7.1)
  line L29 (6.5, 5.1) -> (6.5, 0.1)
  line L30 (8.5, -1.9) -> (19.5, -1.9)
  line L31 (19.5, -1.9) -> (19.5, 5.1)
  line L32 (18.2, -1.4) -> (22.2, -1.4) construction
  line L33 (18.2, -4.4) -> (22.2, -4.4)
  line L34 (22.2, 1.6) -> (18.2, 1.6)
  arc A36 (18.2, 1.6) -> (18.2, -4.4) centre (18.2, -1.4) ccw
  arc A37 (22.2, -4.4) -> (22.2, 1.6) centre (22.2, -1.4) ccw
  line L35 (15.2, -1.4) -> (15.2, -1.9)
  arc A38 (19.5, 5.1) -> (17.5, 7.1) centre (17.5, 5.1) ccw
  arc A39 (8.5, 7.1) -> (6.5, 5.1) centre (8.5, 5.1) ccw
  arc A40 (6.5, 0.1) -> (8.5, -1.9) centre (8.5, 0.1) ccw
  point P0 (0, 0)
  point P1 (6.5, -1.9)
  point P2 (6.5, 7.1)
  point P3 (20.2, -1.4)
  point P4 (19.5, 1.6)
  dimension "d125" = 13
  dimension "d126" = 9
  dimension "d127" = 4
  dimension "d128" = 6
  dimension "d129" = 2
  constraints: 18 end point, 11 point on circle, 10 tangent, 7 point on line, 5 centre point, 3 parallel, 2 equal radius, 2 horizontal, 2 perpendicular, 1 midpoint
  measures "d125" distance of L30.end point (6.5, -1.9)
  measures "d126" distance of point (6.5, -1.9) point (6.5, 7.1)
  measures "d127" distance of L32.start L32.end
  measures "d128" diameter of A37
  measures "d129" radius of A38
extrude "Extrusion19" cut sketch "Sketch20" against normal blind 10 contours L34 A36 L35 L30 A40 L29 A39 L28 A38 L31
fillet "Fillet7" radius 1 2 edges at (-19.5, 1.6, 1) (-15.2, -1.9, 1)
sketch "Sketch21" plane through (0, 0, 0) normal (0, 0, -1) x (-1, 0, 0)
  line L0 (19.5, 5.1) -> (19.5, 2.6) projected
  arc A0 (18.5, 1.6) -> (19.5, 2.6) centre (18.5, 2.6) ccw projected
  line L1 (18.5, 1.6) -> (18.2, 1.6) projected
  arc A1 (18.2, 1.6) -> (15.2235, -1.025) centre (18.2, -1.4) ccw projected
  arc A2 (14.2314, -1.9) -> (15.2235, -1.025) centre (14.2314, -0.9) ccw projected
  line L2 (14.2314, -1.9) -> (8.5, -1.9) projected
  arc A3 (6.5, 0.1) -> (8.5, -1.9) centre (8.5, 0.1) ccw projected
  line L3 (6.5, 0.1) -> (6.5, 5.1) projected
  arc A4 (8.5, 7.1) -> (6.5, 5.1) centre (8.5, 5.1) ccw projected
  line L4 (8.5, 7.1) -> (17.5, 7.1) projected
  arc A5 (19.5, 5.1) -> (17.5, 7.1) centre (17.5, 5.1) ccw projected
  arc A6 (15.2235, -18.775) -> (14.2314, -17.9) centre (14.2314, -18.9) ccw projected
  arc A7 (15.2235, -18.775) -> (18.2, -21.4) centre (18.2, -18.4) ccw projected
  line L5 (18.2, -21.4) -> (18.5, -21.4) projected
  arc A8 (19.5, -22.4) -> (18.5, -21.4) centre (18.5, -22.4) ccw projected
  line L6 (19.5, -22.4) -> (19.5, -24.9) projected
  arc A9 (17.5, -26.9) -> (19.5, -24.9) centre (17.5, -24.9) ccw projected
  line L7 (17.5, -26.9) -> (12.5, -26.9) projected
  arc A10 (10.5, -24.9) -> (12.5, -26.9) centre (12.5, -24.9) ccw projected
  line L8 (10.5, -24.9) -> (10.5, -19.9) projected
  arc A11 (12.5, -17.9) -> (10.5, -19.9) centre (12.5, -19.9) ccw projected
  line L9 (12.5, -17.9) -> (14.2314, -17.9) projected
  line L10 (-16.5, 7.1) -> (-16.5, -26.9) projected
  arc A12 (-16.5, -26.9) -> (-14.5, -28.9) centre (-14.5, -26.9) ccw projected
  line L11 (-14.5, -28.9) -> (19.5, -28.9) projected
  arc A13 (19.5, -28.9) -> (21.5, -26.9) centre (19.5, -26.9) ccw projected
  line L12 (21.5, -26.9) -> (21.5, 7.1) projected
  arc A14 (21.5, 7.1) -> (19.5, 9.1) centre (19.5, 7.1) ccw projected
  line L13 (19.5, 9.1) -> (5.3, 9.1) projected
  line L14 (5.3, 9.1) -> (5.3, 0) projected
  arc A15 (0.7, 0) -> (5.3, 0) centre (3, 0) ccw projected
  line L15 (0.7, 0) -> (0.7, 9.1) projected
  line L16 (0.7, 9.1) -> (-14.5, 9.1) projected
  arc A16 (-14.5, 9.1) -> (-16.5, 7.1) centre (-14.5, 7.1) ccw projected
  line L17 (-3, -3.9) -> (2, -3.9) projected
  arc A17 (2, -5.9) -> (2, -3.9) centre (2, -4.9) ccw projected
  line L18 (2, -5.9) -> (-3, -5.9) projected
  arc A18 (-3, -3.9) -> (-3, -5.9) centre (-3, -4.9) ccw projected
  line L19 (-14.5, 1.1) -> (-14.5, 5.1) projected
  arc A19 (-12.5, 7.1) -> (-14.5, 5.1) centre (-12.5, 5.1) ccw projected
  line L20 (-12.5, 7.1) -> (-2.5, 7.1) projected
  arc A20 (-0.5, 5.1) -> (-2.5, 7.1) centre (-2.5, 5.1) ccw projected
  line L21 (-0.5, 5.1) -> (-0.5, 1.1) projected
  arc A21 (-2.5, -0.9) -> (-0.5, 1.1) centre (-2.5, 1.1) ccw projected
  line L22 (-2.5, -0.9) -> (-12.5, -0.9) projected
  arc A22 (-14.5, 1.1) -> (-12.5, -0.9) centre (-12.5, 1.1) ccw projected
  line L23 (8.6461, -10.4) -> (8.6461, -15.4) projected
  arc A23 (6.6461, -15.4) -> (8.6461, -15.4) centre (7.6461, -15.4) ccw projected
  line L24 (6.6461, -15.4) -> (6.6461, -10.4) projected
  arc A24 (8.6461, -10.4) -> (6.6461, -10.4) centre (7.6461, -10.4) ccw projected
  circle A25 centre (2.5, -9.9) radius 1.5 projected
  line L25 (-12.5, -17.9) -> (-7.5, -17.9) projected
  arc A26 (-5.5, -19.9) -> (-7.5, -17.9) centre (-7.5, -19.9) ccw projected
  line L26 (-5.5, -19.9) -> (-5.5, -24.9) projected
  arc A27 (-7.5, -26.9) -> (-5.5, -24.9) centre (-7.5, -24.9) ccw projected
  line L27 (-7.5, -26.9) -> (-12.5, -26.9) projected
  arc A28 (-14.5, -24.9) -> (-12.5, -26.9) centre (-12.5, -24.9) ccw projected
  line L28 (-14.5, -24.9) -> (-14.5, -19.9) projected
  arc A29 (-12.5, -17.9) -> (-14.5, -19.9) centre (-12.5, -19.9) ccw projected
  circle A30 centre (18.2, -1.4) radius 0.95 projected
  circle A31 centre (18.2, -18.4) radius 0.95 projected
  circle A32 centre (-3, -24.8) radius 0.8 projected
  circle A33 centre (2.5, -14.9) radius 0.8 projected
  circle A34 centre (-12.4, -15.4) radius 0.8 projected
  circle A35 centre (-12.4, -4.4) radius 0.8 projected
  circle A36 centre (-2.5, -9.9) radius 0.8 projected
  circle A37 centre (8, -24.8) radius 0.8 projected
  line L29 (-5.45, -6.9) -> (-5.45, -12.9) projected
  arc A38 (-9.45, -12.9) -> (-5.45, -12.9) centre (-7.45, -12.9) ccw projected
  line L30 (-9.45, -12.9) -> (-9.45, -6.9) projected
  arc A39 (-5.45, -6.9) -> (-9.45, -6.9) centre (-7.45, -6.9) ccw projected
  line L31 (-0.5, -17.85) -> (5.5, -17.85) projected
  arc A40 (5.5, -21.85) -> (5.5, -17.85) centre (5.5, -19.85) ccw projected
  line L32 (5.5, -21.85) -> (-0.5, -21.85) projected
  arc A41 (-0.5, -17.85) -> (-0.5, -21.85) centre (-0.5, -19.85) ccw projected
  line L33 (18.2, -1.4) -> (18.2, -18.4)
  line L34 (18.2, -9.9) -> (14.7, -9.9)
  line L35 (12.7, -4.9) -> (16.7, -4.9)
  line L36 (18.7, -6.9) -> (18.7, -12.9)
  line L37 (16.7, -14.9) -> (12.7, -14.9)
  line L38 (10.7, -12.9) -> (10.7, -6.9)
  line L39 (10.7, -4.9) -> (18.7, -14.9) construction
  line L40 (18.7, -4.9) -> (10.7, -14.9) construction
  arc A42 (18.7, -6.9) -> (16.7, -4.9) centre (16.7, -6.9) ccw
  arc A43 (16.7, -14.9) -> (18.7, -12.9) centre (16.7, -12.9) ccw
  arc A44 (10.7, -12.9) -> (12.7, -14.9) centre (12.7, -12.9) ccw
  arc A45 (12.7, -4.9) -> (10.7, -6.9) centre (12.7, -6.9) ccw
  point P0 (0, 0)
  dimension "d133" = 3.5
  dimension "d134" = 8
  dimension "d135" = 10
  dimension "d136" = 2
  constraints: 16 end point, 8 point on circle, 8 point on line, 8 tangent, 4 centre point, 3 equal radius, 3 midpoint, 2 horizontal, 2 parallel, 1 perpendicular, 1 vertical
  measures "d133" distance of L34.start L34.end
  measures "d134" distance of L39.start L40.start
  measures "d135" distance of L40.start L39.end
  measures "d136" radius of A42
extrude "Extrusion20" cut sketch "Sketch21" against normal blind 10 contours A42 L36 A43 L33 | L33 A43 L37 A44 L38 A45 L35 A42
fillet "Fillet8" radius 1 9 edges at (-20.9142, 8.5142, 0) (-12.4, 9.1, 0) (-20.9142, -28.3142, 0) (-2.5, -28.9, 0) (15.9142, -28.3142, 0) (16.5, -9.9, 0) (15.9142, 8.5142, 0) (6.9, 9.1, 0) (-21.5, -9.9, 0)
fillet "Fillet9" radius 1 1 edges at (-3, 9.1, -2.5)
fillet "Fillet10" radius 1 9 edges at (-0.7, 8.8071, -0.2929) (-0.7, 9.1, -3) (-0.7, 9.1, -1.7499) (-3, -2.3, 0) (-5.3, 4.05, 0) (-5.3, 8.8071, -0.2929) (-5.3, 9.1, -3) (-5.3, 9.1, -1.7499) (-0.7, 4.05, 0)
body "Solid1"
